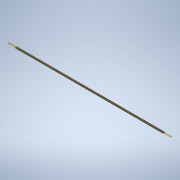
# Autodesk Inventor part: fuselage_rod
Saved by Autodesk Inventor 2021 (Build 250183000, 183)
## iProperties
Created: 2020-11-15
Part Number: fuselage_rod
Material: CFRP
Document SubType Name: Modeling
Designer: Paco
Density: 1.43 g/cm^3
Appearance: Carbon Fiber
Mass: 9.438 g
Surface Area: 132.24 cm^2
Volume: 6.6 cm^3
Author: Paco
Autodesk Inventor part; units mm, degrees
ref_plane "YZ Plane" through (0, 0, 0) normal (1, 0, 0) x (0, 1, 0)
sketch "Sketch1" plane through (0, 0, 0) normal (1, 0, 0) x (0, 1, 0)
  line L0 (-2, 2) -> (2, 2)
  line L1 (2, 2) -> (2, -2)
  line L2 (2, -2) -> (-2, -2)
  line L3 (-2, -2) -> (-2, 2)
  line L4 (-2, 2) -> (2, -2) construction
  line L5 (2, 2) -> (-2, -2) construction
  line L6 (1, 1) -> (-1, 1)
  line L7 (-1, 1) -> (-1, -1)
  line L8 (-1, -1) -> (1, -1)
  line L9 (1, -1) -> (1, 1)
  line L10 (1, 1) -> (-1, -1) construction
  line L11 (-1, 1) -> (1, -1) construction
  point P0 (0, 0)
  point P1 (0, 0)
  point P2 (0, 0)
  dimension "d8" = 4
  dimension "d9" = 4
  dimension "d10" = 2
  dimension "d11" = 2
  constraints: 24 end point, 5 midpoint, 4 parallel, 2 horizontal, 2 perpendicular, 1 coincident, 1 point on line, 1 other
  measures "d8" distance of L0.end L1.end
  measures "d9" distance of L1.end L2.end
  measures "d10" distance of L7.end L8.end
  measures "d11" distance of L8.end L6.start
extrude "Extrusion1" add sketch "Sketch1" along normal blind 550
body "Solid1"
